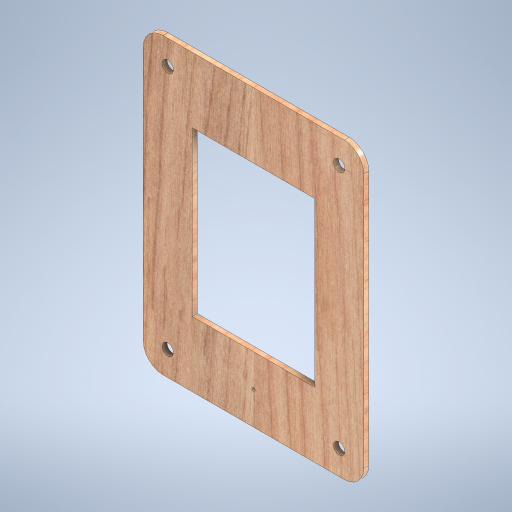
# Autodesk Inventor part: TapaBC
Saved by Autodesk Inventor 2023.1 (Build 271208000, 208)
## iProperties
Created: 2022-11-11
Part Number: TapaBC
Material: MDF Medium Density Fiberboard
Document SubType Name: Modeling
Designer: Daniel Peña
Density: 0.8 g/cm^3
Appearance: Birch - Natural Polished
Author: Daniel Peña
Autodesk Inventor part; units mm, degrees
ref_plane "YZ Plane" through (0, 0, 0) normal (1, 0, 0) x (0, 1, 0)
ref_plane "XZ Plane" through (0, 0, 0) normal (0, 1, 0) x (-1, 0, 0)
ref_plane "XY Plane" through (0, 0, 0) normal (0, 0, 1) x (1, 0, 0)
sketch "Sketch1" plane through (0, 0, 0) normal (0, 0, 1) x (1, 0, 0)
  line L0 (-55.5, 90) -> (55.5, 90)
  line L1 (67.5, 78) -> (67.5, -78)
  line L2 (55.5, -90) -> (-55.5, -90)
  line L3 (-67.5, -78) -> (-67.5, 78)
  line L4 (-37.5, 50) -> (37.5, 50)
  line L5 (37.5, 50) -> (37.5, -50)
  line L6 (37.5, -50) -> (-37.5, -50)
  line L7 (-37.5, -50) -> (-37.5, 50)
  arc A0 (-55.5, 90) -> (-67.5, 78) centre (-55.5, 78) ccw
  arc A1 (67.5, 78) -> (55.5, 90) centre (55.5, 78) ccw
  arc A2 (55.5, -90) -> (67.5, -78) centre (55.5, -78) ccw
  arc A3 (-67.5, -78) -> (-55.5, -90) centre (-55.5, -78) ccw
  point P0 (0, 0)
  point P1 (-67.5, 90)
  point P2 (67.5, -90)
  point P3 (67.5, 90)
  point P4 (-67.5, -90)
  dimension "d0" = 180
  dimension "d2" = 100
  dimension "d3" = 40
  dimension "d4" = 40
  dimension "d7" = 30
  dimension "d8" = 30
  dimension "d10" = 75
  dimension "d11" = 12
  dimension "d21" = 37.5
  dimension "d22" = 50
  constraints: 16 end point, 8 point on circle, 8 point on line, 8 tangent, 4 centre point, 4 parallel, 3 equal radius, 2 horizontal, 2 perpendicular
  measures "d0" distance of point (-67.5, -90) point (-67.5, 90)
  measures "d2" distance between parallel lines of L6 L4
  measures "d3" distance between parallel lines of L0 L4
  measures "d4" distance between parallel lines of L2 L6
  measures "d7" distance between parallel lines of L7 L3
  measures "d8" distance between parallel lines of L1 L5
  measures "d10" distance between parallel lines of L5 L7
  measures "d11" radius of A0
  measures "d21" distance from line of point (0, 0) L7
  measures "d22" distance from line of L4 point (0, 0)
extrude "Extrusion1" add sketch "Sketch1" along normal blind 3
sketch "Sketch3" plane through (0, 0, 3) normal (0, 0, 1) x (1, 0, 0)
  line L0 (55.5, 90) -> (-55.5, 90) construction
  line L1 (0, 90) -> (0, -90) construction
  line L2 (-55.5, -90) -> (55.5, -90) construction
  line L3 (-67.5, 78) -> (-67.5, -78) construction
  line L4 (-67.5, 0) -> (67.5, 0) construction
  line L5 (67.5, -78) -> (67.5, 78) construction
  point P0 (0, 0)
  point P1 (-52.5, 75)
  point P2 (52.5, 75)
  point P3 (52.5, -75)
  point P4 (-52.5, -75)
  dimension "d12" = 15
  dimension "d13" = 15
  constraints: 4 end point, 4 midpoint, 3 symmetric about line
  measures "d12" distance from line of L3 point (-52.5, 75)
  measures "d13" distance from line of point (-52.5, 75) L0
hole "Hole1" at (-52.5, 75, 3) at (52.5, 75, 3) at (52.5, -75, 3) at (-52.5, -75, 3) direction (0, 0, -1) diameter 7 end through all
sketch "Sketch4" plane through (0, 0, 3) normal (0, 0, 1) x (1, 0, 0)
  line L0 (-55.5, -90) -> (55.5, -90) projected
  line L1 (67.5, -78) -> (67.5, 78) projected
  point P0 (0, 0)
  point P1 (0, -70)
  dimension "d23" = 20
  dimension "d24" = 67.5
  measures "d23" distance from line of L0 point (0, -70)
  measures "d24" distance from line of L1 point (0, -70)
hole "Hole2" at (0, -70, 3) direction (0, 0, -1) diameter 2 depth 1
equation "\"d3\" = d4"
equation "\"d8\" = d7"
equation "\"d21\" = 0.5 * d10"
equation "\"d22\" = 0.5 * d2"
body "Solid1"
